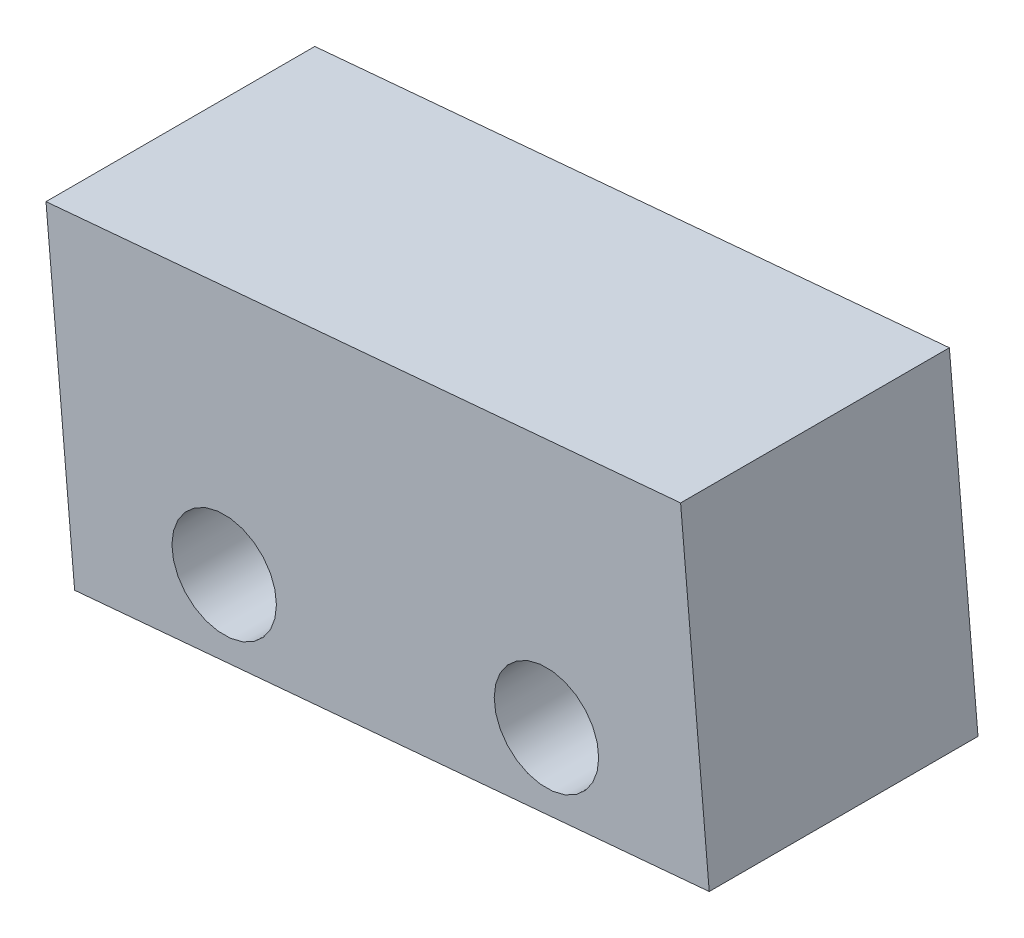
# Autodesk Inventor part: Microswitch_Fixture
Saved by Autodesk Inventor 2016 (Build 200138000, 138)
## iProperties
Created: 2015-07-29
Part Number: Microswitch_Fixture
Material: Generic
Document SubType Name: Modeling
Designer: 3DPrinterUser
Density: 1 g/cm^3
Appearance: Magenta
Author: 3DPrinterUser
Autodesk Inventor part; units mm, degrees
ref_plane "YZ Plane" through (0, 0, 0) normal (1, 0, 0) x (0, 1, 0)
ref_plane "XZ Plane" through (0, 0, 0) normal (0, 1, 0) x (-1, 0, 0)
ref_plane "XY Plane" through (0, 0, 0) normal (0, 0, 1) x (1, 0, 0)
derived "Transmission.ipt"
sketch "Sketch1" plane through (0, 0, 0) normal (0, 0, 1) x (1, 0, 0)
  line L0 (51.4447, -24.8242) -> (52.0198, -31.2987) projected
  line L1 (38.6949, -25.9568) -> (56.6243, -24.3641) projected
  line L2 (39.27, -32.4313) -> (38.6949, -25.9568) projected
  line L3 (52.0198, -31.2987) -> (39.27, -32.4313) projected
  line L4 (51.4447, -24.8242) -> (38.6949, -25.9568)
  circle A0 centre (42.275, -30.6584) radius 1.05 projected
  circle A1 centre (48.7495, -30.0833) radius 1.05 projected
  point P0 (0, 0)
  constraints: 2 end point, 1 collinear
extrude "Extrusion1" add sketch "Sketch1" along normal blind 5.4
body "Solid1"
